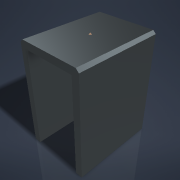
# Autodesk Inventor part: magnetGuide
Saved by Autodesk Inventor 2022 (Build 260153070, 153G)
## iProperties
Created: 2022-02-03
Part Number: magnetGuide
Material: Железо, мягкое
Document SubType Name: Обычные детали
Designer: kalugin_a
Density: 7.15 g/cm^3
Appearance: Чугун серый
Sheet Metal Width: 0,000 мм
Sheet Metal Length: 0,000 мм
Sheet Metal Area: 0,000 мм^2
Sheet Metal Rule: По умолчанию_мм
Author: kalugin_a
Autodesk Inventor part; units mm, degrees
ref_plane "YZ Plane" through (0, 0, 0) normal (1, 0, 0) x (0, 1, 0)
ref_plane "XZ Plane" through (0, 0, 0) normal (0, 1, 0) x (-1, 0, 0)
sketch "Эскиз1" plane through (0, 0, 0) normal (0, 1, 0) x (-1, 0, 0)
  line L0 (-23, 30) -> (23, 30)
  line L1 (23, 30) -> (23, -30)
  line L2 (23, -30) -> (-23, -30)
  line L3 (-23, -30) -> (-23, 30)
  line L4 (-18, 30) -> (18, 30)
  line L5 (18, 30) -> (18, -30)
  line L6 (18, -30) -> (-18, -30)
  line L7 (-18, -30) -> (-18, 30)
  point P0 (0, 0)
  point P1 (-18, 30)
  point P2 (-18, -30)
  dimension "d0" = 46
  dimension "d2" = 36
  dimension "d3" = 60
  dimension "d14" = 5
  constraints: 16 end point, 4 parallel, 2 horizontal, 2 perpendicular
  measures "d0" distance of L1.end L2.end
  measures "d2" distance of L5.end L6.end
  measures "d3" distance of L4.end L5.end
  measures "d14" distance of L4.end L0.end
extrude "Выдавливание3" add sketch "Эскиз1" against normal blind 5 contours L0 L5 L2 L7
extrude "Выдавливание4" add sketch "Эскиз1" against normal blind 75 contours L0 L7 L2 L3 | L0 L1 L2 L5
ref_plane "РабПлоскость5" through (0, -2.5, 0) normal (0, 1, 0) x (-1, 0, 0)
sketch "Эскиз3" plane through (0, -75, 0) normal (0, -1, 0) x (1, 0, 0)
  line L0 (-18, 30) -> (-23, 30) projected
  line L1 (-23, -30) -> (-18, -30) projected
  point P0 (0, 0)
  point P1 (-20.322, 15)
  point P2 (-20.4927, -15)
  point P3 (20.6897, -15.1643)
  dimension "d59" = 15
  dimension "d60" = 15
  measures "d59" distance from line of L0 point (-20.322, 15)
  measures "d60" distance from line of L1 point (-20.493, -15)
sketch "Эскиз4" plane through (0, -75, 0) normal (0, -1, 0) x (1, 0, 0)
  line L0 (-23, -30) -> (-18, -30) projected
  line L1 (-18, -30) -> (-18, 30) projected
  point P0 (0, 0)
  point P1 (-20.5, -15)
  dimension "d43" = 15
  dimension "d44" = 2.5
  measures "d43" distance from line of L0 point (-20.5, -15)
  measures "d44" distance from line of L1 point (-20.5, -15)
hole "Отверстие3" at (-20.5, -75, -15) direction (0, 1, 0) diameter 2.459 depth 8.8 tip angle 118 thread size "M3x0.5" class "6H" standard "ISO Metric profile"
hole "Отверстие4" at (-20.322, -75, 15) direction (0, 1, 0) diameter 2.459 depth 8.8 tip angle 118 thread size "M3x0.5" class "6H" standard "ISO Metric profile"
sketch "Эскиз5" plane through (0, -75, 0) normal (0, -1, 0) x (1, 0, 0)
  circle A0 centre (-20.322, 15) radius 1.2295 construction
  circle A1 centre (-20.5, -15) radius 1.2295 projected
  point P0 (0, 0)
  point P1 (20.4588, 15)
  point P2 (20.4588, -15)
hole "Отверстие5" at (20.4588, -75, 15) at (20.4588, -75, -15) direction (0, 1, 0) diameter 2.459 depth 8.8 tip angle 118 thread size "M3x0.5" class "6H" standard "ISO Metric profile"
sketch "Эскиз9" plane through (23, 0, -30) normal (0, 0, -1) x (-1, 0, 0)
  point P0 (23, 0)
  point P1 (23.0428, -2.5128)
hole "Отверстие7" at (-0.0428, -2.5128, -30) direction (0, 0, 1) diameter 2.459 depth 8.8 tip angle 118 thread size "M3x0.5" class "6H" standard "ISO Metric profile"
sketch "Эскиз8" plane through (23, 0, -30) normal (0, 0, -1) x (-1, 0, 0)
  line L0 (0, 0) -> (0, -75) projected
  line L1 (0, 0) -> (46, 0) construction
  line L2 (46, 0) -> (46, -75) projected
  line L3 (5, -5) -> (5, -75) projected
  line L4 (3.7707, -75) -> (1.3117, -75) projected
  line L5 (2.5, -75) -> (2.5, 0) construction
  line L6 (46, 0) -> (46, -75) construction
  line L7 (46, -2.5) -> (0, -2.5) construction
  line L8 (44.7295, -75) -> (42.2705, -75) construction
  line L9 (43.5, -75) -> (43.5, 0) construction
  line L10 (2.5, -20) -> (43.5, -20) construction
  line L11 (43.5, -20) -> (43.5, -55) construction
  line L12 (43.5, -55) -> (2.5, -55) construction
  line L13 (2.5, -55) -> (2.5, -20) construction
  line L14 (0, -75) -> (0, 0) projected
  line L15 (0, 0) -> (46, 0) projected
  line L16 (46, 0) -> (46, -75) projected
  line L17 (46, -75) -> (41, -75) projected
  line L18 (41, -75) -> (41, -5) projected
  line L19 (41, -5) -> (5, -5) projected
  line L20 (5, -5) -> (5, -75) projected
  line L21 (5, -75) -> (0, -75) projected
  circle A0 centre (23.0428, -2.5128) radius 1.2295 projected
  point P0 (23, 0)
  dimension "d76" = 5
  dimension "d84" = 35
  constraints: 14 end point, 7 point on line, 4 perpendicular, 3 coincident, 2 parallel, 1 horizontal, 1 midpoint
  measures "d76" distance between parallel lines of L0 L3
  measures "d84" distance of L10.end L11.end
hole "Отверстие9" at (20.5, -55, -30) direction (0, 0, 1) diameter 2.459 depth 8.8 tip angle 118 thread size "M3x0.5" class "6H" standard "ISO Metric profile"
hole "Отверстие10" at (-20.5, -55, -30) at (20.5, -20, -30) direction (0, 0, 1) diameter 2.459 depth 8.8 tip angle 118 thread size "M3x0.5" class "6H" standard "ISO Metric profile"
hole "Отверстие11" at (-20.5, -20, -30) direction (0, 0, 1) diameter 2.459 depth 8.8 tip angle 118 thread size "M3x0.5" class "6H" standard "ISO Metric profile"
chamfer "Фаска1" distance 2 angle 45 2 edges at (23, 0, 0) (-23, 0, 0)
equation "\"Радиус_гибки\" = Толщина"
equation "\"Ширина_просечки\" = Толщина"
equation "\"Глубина_просечки\" = 0.5 * Толщина"
equation "\"Радиус_перехода\" = Радиус_гибки"
equation "\"Радиус_Якоби\" = Радиус_гибки"
equation "\"Размер_зазора\" = Толщина"
equation "\"Толщина\" = 5"
